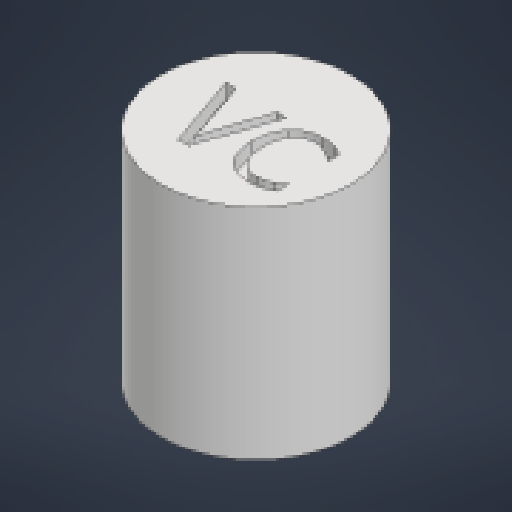
# Autodesk Inventor part: VialCarousel
Saved by Autodesk Inventor 2024.2 (Build 282272000, 272)
## iProperties
Created: 2024-10-04
Part Number: VialCarousel
Material: Generic
Document SubType Name: Modeling
Designer: jerem
Density: 1 g/cm^3
Appearance: Default
Author: jerem
Autodesk Inventor part; units mm, degrees
ref_plane "YZ Plane" through (0, 0, 0) normal (1, 0, 0) x (0, 1, 0)
ref_plane "XZ Plane" through (0, 0, 0) normal (0, 1, 0) x (-1, 0, 0)
ref_plane "XY Plane" through (0, 0, 0) normal (0, 0, 1) x (1, 0, 0)
sketch "Sketch1" plane through (0, 0, 0) normal (0, 1, 0) x (-1, 0, 0)
  circle A0 centre (0, 0) radius 65
  line L0 (0, 0) -> (0, -25) construction
  circle A1 centre (0, -25) radius 11.5 construction
  circle A2 centre (21.6506, -12.5) radius 11.5 construction
  circle A3 centre (21.6506, 12.5) radius 11.5 construction
  circle A4 centre (0, 25) radius 11.5 construction
  circle A5 centre (-21.6506, 12.5) radius 11.5 construction
  circle A6 centre (-21.6506, -12.5) radius 11.5 construction
  line L1 (0, 0) -> (-21.6506, 37.5) construction
  circle A7 centre (-21.6506, 37.5) radius 11.5 construction
  circle A8 centre (-43.3013, 0) radius 11.5 construction
  circle A9 centre (-21.6506, -37.5) radius 11.5 construction
  circle A10 centre (21.6506, -37.5) radius 11.5 construction
  circle A11 centre (43.3013, 0) radius 11.5 construction
  circle A12 centre (21.6506, 37.5) radius 11.5 construction
  circle A13 centre (0, 50) radius 11.5 construction
  circle A14 centre (-43.3013, 25) radius 11.5 construction
  circle A15 centre (-43.3013, -25) radius 11.5 construction
  circle A16 centre (0, -50) radius 11.5 construction
  circle A17 centre (43.3013, -25) radius 11.5 construction
  circle A18 centre (43.3013, 25) radius 11.5 construction
  dimension "d0" = 130
  dimension "d5" = 25
  dimension "d6" = 23
  dimension "d9" = 360
  dimension "d11" = 23
  dimension "d13" = 150
  dimension "d16" = 360
  dimension "d18" = 25
  dimension "d19" = 25
  dimension "d20" = 25
  dimension "d21" = 25
  dimension "d22" = 23
  dimension "d25" = 360
  constraints: 19 centre point, 4 end point, 3 coincident, 1 vertical, 39 other
  measures "d0" diameter of A0
  measures "d5" distance of L0.start L0.end
  measures "d6" diameter of A1
  measures "d11" diameter of A7
  measures "d13" angle of L1 L0
  measures "d18" distance of A12.centre A4.centre
  measures "d19" distance of A4.centre A3.centre
  measures "d20" distance of A4.centre A13.centre
  measures "d21" distance of A12.centre A13.centre
  measures "d22" diameter of A13
extrude "Extrusion1" add sketch "Sketch1" along normal blind 150
sketch "Sketch2" plane through (0, 150, 0) normal (0, 1, 0) x (1, 0, 0)
  line L0 (-37.7255, 18.2555) -> (-21.2587, 18.2555) construction
  line L1 (-21.2587, 18.2555) -> (-21.2587, 7.8989) construction
  line L2 (-21.2587, 7.8989) -> (-37.7255, 7.8989) construction
  line L3 (-37.7255, 7.8989) -> (-37.7255, 18.2555) construction
  line L4 (3.6035, 17.3641) -> (-13.6169, -32.6359)
  line L5 (-13.6169, -32.6359) -> (-20.7887, -32.6359)
  line L6 (-20.7887, -32.6359) -> (-38.0091, 17.3641)
  line L7 (-38.0091, 17.3641) -> (-30.8779, 17.3641)
  line L8 (-30.8779, 17.3641) -> (-17.0205, -24.1675)
  line L9 (-17.0205, -24.1675) -> (-3.1631, 17.3641)
  line L10 (-3.1631, 17.3641) -> (3.6035, 17.3641)
  spline S0 degree 2 poles (27.9147, -33.5273) (23.0524, -33.5273) (14.8272, -30.2453) (11.8288, -26.9633) knots 0 0 0 1 2 2 2
  spline S1 degree 2 poles (11.8288, -26.9633) (8.8304, -23.7218) (5.5484, -13.9973) (5.5484, -7.6764) knots 0 0 0 1 2 2 2
  spline S2 degree 2 poles (5.5484, -7.6764) (5.5484, -1.396) (8.7494, 7.9232) (11.7883, 11.3673) knots 0 0 0 1 2 2 2
  spline S3 degree 2 poles (11.7883, 11.3673) (14.7866, 14.7304) (22.9714, 18.2555) (28.0362, 18.2555) knots 0 0 0 1 2 2 2
  spline S4 degree 2 poles (28.0362, 18.2555) (30.5484, 18.2555) (34.9649, 17.5262) (36.8288, 16.9589) knots 0 0 0 1 2 2 2
  spline S5 degree 2 poles (36.8288, 16.9589) (38.4495, 16.4322) (41.8126, 14.933) (43.4738, 14.0416) knots 0 0 0 1 2 2 2
  line L11 (43.4738, 14.0416) -> (43.4738, 6.0189)
  line L12 (43.4738, 6.0189) -> (42.9471, 6.0189)
  spline S6 degree 2 poles (42.9471, 6.0189) (42.0557, 6.8292) (39.3004, 9.0983) (37.315, 10.1923) knots 0 0 0 1 2 2 2
  spline S7 degree 2 poles (37.315, 10.1923) (35.4106, 11.2458) (30.9131, 12.5829) (27.9957, 12.5829) knots 0 0 0 1 2 2 2
  spline S8 degree 2 poles (27.9957, 12.5829) (24.7947, 12.5829) (19.0816, 9.9492) (16.9341, 7.437) knots 0 0 0 1 2 2 2
  spline S9 degree 2 poles (16.9341, 7.437) (14.8272, 4.8843) (12.4771, -2.8547) (12.4771, -7.6764) knots 0 0 0 1 2 2 2
  spline S10 degree 2 poles (12.4771, -7.6764) (12.4771, -12.8223) (14.9487, -20.2372) (17.0962, -22.7899) knots 0 0 0 1 2 2 2
  spline S11 degree 2 poles (17.0962, -22.7899) (19.2032, -25.2615) (24.8353, -27.7737) (27.9957, -27.7737) knots 0 0 0 1 2 2 2
  spline S12 degree 2 poles (27.9957, -27.7737) (30.8725, -27.7737) (35.7753, -26.3555) (37.6797, -25.302) knots 0 0 0 1 2 2 2
  spline S13 degree 2 poles (37.6797, -25.302) (39.503, -24.2486) (42.2178, -22.0606) (42.9876, -21.2907) knots 0 0 0 1 2 2 2
  line L13 (42.9876, -21.2907) -> (43.4738, -21.2907)
  line L14 (43.4738, -21.2907) -> (43.4738, -29.2324)
  spline S14 degree 2 poles (43.4738, -29.2324) (41.8126, -30.0022) (38.8952, -31.4204) (36.8288, -32.0687) knots 0 0 0 1 2 2 2
  spline S15 degree 2 poles (36.8288, -32.0687) (34.6408, -32.798) (30.9131, -33.5273) (27.9147, -33.5273) knots 0 0 0 1 2 2 2
  point P0 (0, 0)
  constraints: 2 other
extrude "Extrusion2" cut sketch "Sketch2" against normal blind 10
equation "\"d11\" = d6"
equation "\"d21\" = d19"
equation "\"d22\" = d6"
body "Solid1"
